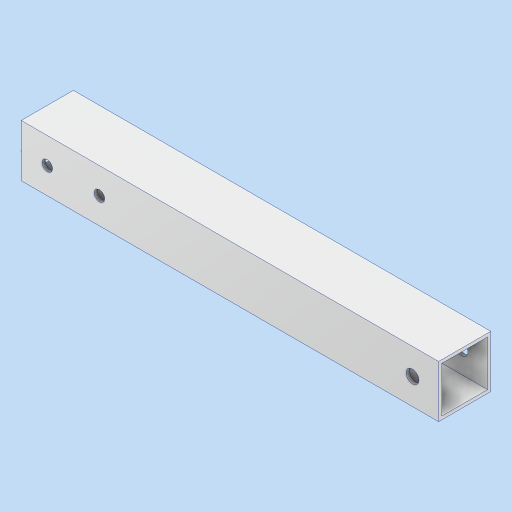
# Autodesk Inventor part: Part1-17-7.9
Saved by Autodesk Inventor 2024 (Build 280153000, 153)
## iProperties
Created: 2023-03-16
Part Number: Part1-17-7.9
Material: Aluminum 6061
Document SubType Name: Modeling
Designer: mvp5338
Density: 2.7 g/cm^3
Appearance: Aluminum - Flat
Author: mvp5338
Autodesk Inventor part; units mm, degrees
ref_plane "YZ Plane" through (0, 0, 0) normal (1, 0, 0) x (0, 1, 0)
ref_plane "XZ Plane" through (0, 0, 0) normal (0, 1, 0) x (-1, 0, 0)
ref_plane "XY Plane" through (0, 0, 0) normal (0, 0, 1) x (1, 0, 0)
sketch "Sketch1" plane through (0, 0, 0) normal (1, 0, 0) x (0, 1, 0)
  line L0 (12.7, 12.2788) -> (-12.7, 12.2788)
  line L1 (-12.7, 12.2788) -> (-12.7, -13.1212)
  line L2 (-12.7, -13.1212) -> (12.7, -13.1212)
  line L3 (12.7, -13.1212) -> (12.7, 12.2788)
  line L4 (0, 32.4321) -> (0, -31.5519)
  line L5 (24.3369, 0) -> (-19.9975, 0)
  point P0 (0, 0)
  dimension "d0" = 25.4
  constraints: 12 end point, 2 horizontal, 2 parallel, 2 perpendicular, 1 vertical, 1 other
  measures "d0" distance of L2.end L0.start
extrude "Extrusion1" add sketch "Sketch1" along normal blind 203.2
sketch "Sketch3" plane through (203.2, 0, 0) normal (1, 0, 0) x (0, 0, -1)
  line L0 (-10.6786, 11.1125) -> (11.521, 11.1125)
  line L1 (11.521, 11.1125) -> (11.521, -11.0998)
  line L2 (11.521, -11.0998) -> (-10.6786, -11.0998)
  line L3 (-10.6786, -11.0998) -> (-10.6786, 11.1125)
  line L4 (13.1212, 12.7) -> (-12.2788, 12.7) projected
  line L5 (-12.2788, 12.7) -> (-12.2788, -12.7) projected
  line L6 (13.1212, -12.7) -> (13.1212, 12.7) projected
  line L7 (-12.2788, -12.7) -> (13.1212, -12.7) projected
  point P0 (0, 0)
  dimension "d5" = 1.5875
  dimension "d6" = 1.6002
  dimension "d7" = 1.6002
  dimension "d8" = 1.6002
  constraints: 8 end point, 2 parallel, 1 horizontal, 1 perpendicular
  measures "d5" distance between parallel lines of L4 L0
  measures "d6" distance between parallel lines of L5 L3
  measures "d7" distance between parallel lines of L6 L1
  measures "d8" distance between parallel lines of L7 L2
extrude "Extrusion2" cut sketch "Sketch3" against normal blind 279.4 contours L0 L1 L2 L3
sketch "Sketch4" plane through (0, -12.7, 12.2788) normal (0, 0, 1) x (1, 0, 0)
  circle A0 centre (190.5, 12.7) radius 3.175
  line L0 (203.2, 25.4) -> (203.2, 0) projected
  circle A1 centre (12.7, 12.7) radius 2.5781
  circle A2 centre (38.1, 12.7) radius 2.5781
  line L1 (0, 25.4) -> (203.2, 25.4) projected
  line L2 (0, 25.4) -> (0, 0) projected
  point P0 (0, 12.7)
  dimension "d11" = 6.35
  dimension "d12" = 12.7
  dimension "d15" = 5.1562
  dimension "d16" = 5.1562
  dimension "d17" = 25.4
  dimension "d18" = 12.7
  dimension "d19" = 12.7
  dimension "d20" = 12.7
  constraints: 3 centre point
  measures "d11" diameter of A0
  measures "d12" distance from line of L0 A0.centre
  measures "d15" diameter of A1
  measures "d16" diameter of A2
  measures "d17" distance of A2.centre A1.centre
  measures "d18" distance from line of L1 A1.centre
  measures "d19" distance from line of L1 A2.centre
  measures "d20" distance from line of L2 A1.centre
extrude "Extrusion3" cut sketch "Sketch4" against normal blind 25.4
sketch "Sketch5" plane through (0, -12.7, 12.2788) normal (0, 0, 1) x (1, 0, 0)
  point P0 (0, 12.7)
equation "\"d19\" = d18"
body "Solid1"
